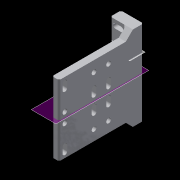
# Autodesk Inventor part: AXTS
Saved by Autodesk Inventor 2016 (Build 200138000, 138)
## iProperties
Created: 2017-07-16
Part Number: AXTS
Material: PC/ABS Plastic
Document SubType Name: Modeling
Designer: ludwi
Density: 0.357273 g/cm^3
Appearance: Smooth - White
Author: ludwi
Autodesk Inventor part; units mm, degrees
ref_plane "YZ Plane" through (0, 0, 0) normal (1, 0, 0) x (0, 1, 0)
ref_plane "XZ Plane" through (0, 0, 0) normal (0, 1, 0) x (-1, 0, 0)
ref_plane "XY Plane" through (0, 0, 0) normal (0, 0, 1) x (1, 0, 0)
sketch "Sketch1" plane through (0, 0, 0) normal (0, 0, 1) x (1, 0, 0)
  line L0 (0, 0) -> (32, 0)
  line L1 (32, 0) -> (32, -120)
  line L2 (32, -120) -> (22, -120)
  line L3 (22, -120) -> (22, -15)
  line L4 (22, -15) -> (0, -15)
  line L5 (0, -15) -> (0, 0)
  dimension "d3" = 120
  dimension "d4" = 10
  dimension "d5" = 22
  dimension "d8" = 15
  constraints: 12 end point, 4 perpendicular, 1 horizontal, 1 vertical
  measures "d3" distance of L0.end L1.end
  measures "d4" distance of L1.end L2.end
  measures "d5" horizontal distance of L0.start L2.end
  measures "d8" distance of L4.end L0.start
extrude "Extrusion1" add sketch "Sketch1" against normal blind 120
sketch "Sketch3" plane through (0, -15, 0) normal (-1, 0, 0) x (0, 0, 1)
  line L0 (-110, -97.8692) -> (-110, 18.1308) construction
  line L1 (-10, 18.1308) -> (-10, -97.8692) construction
  line L2 (-25, 8.9558) -> (-17, 8.9558) construction
  arc A0 (-17, 8.9558) -> (-17, 15.0558) centre (-17, 12.0058) ccw construction
  line L3 (-17, 15.0558) -> (-25, 15.0558) construction
  arc A1 (-25, 15.0558) -> (-25, 8.9558) centre (-25, 12.0058) ccw construction
  line L4 (-25, -94.7942) -> (-17, -94.7942) construction
  arc A2 (-17, -94.7942) -> (-17, -88.6942) centre (-17, -91.7442) ccw construction
  line L5 (-17, -88.6942) -> (-25, -88.6942) construction
  arc A3 (-25, -88.6942) -> (-25, -94.7942) centre (-25, -91.7442) ccw construction
  circle A4 centre (-25, -50.2442) radius 3.05 construction
  circle A5 centre (-25, -29.4942) radius 3.05 construction
  circle A6 centre (-95, -29.4942) radius 3.05 construction
  circle A7 centre (-95, -50.2442) radius 3.05 construction
  line L6 (-95, 15.0558) -> (-103, 15.0558) construction
  arc A8 (-103, 15.0558) -> (-103, 8.9558) centre (-103, 12.0058) ccw construction
  line L7 (-103, 8.9558) -> (-95, 8.9558) construction
  arc A9 (-95, 8.9558) -> (-95, 15.0558) centre (-95, 12.0058) ccw construction
  circle A10 centre (-67.125, 12.0058) radius 3.05 construction
  line L8 (-52.875, -32.5442) -> (-44.875, -32.5442) construction
  arc A11 (-44.875, -32.5442) -> (-44.875, -26.4442) centre (-44.875, -29.4942) ccw construction
  line L9 (-44.875, -26.4442) -> (-52.875, -26.4442) construction
  arc A12 (-52.875, -26.4442) -> (-52.875, -32.5442) centre (-52.875, -29.4942) ccw construction
  circle A13 centre (-52.875, -91.7442) radius 3.05 construction
  circle A14 centre (-52.875, 12.0058) radius 3.05 construction
  line L10 (-52.875, -53.2942) -> (-44.875, -53.2942) construction
  arc A15 (-44.875, -53.2942) -> (-44.875, -47.1942) centre (-44.875, -50.2442) ccw construction
  line L11 (-44.875, -47.1942) -> (-52.875, -47.1942) construction
  arc A16 (-52.875, -47.1942) -> (-52.875, -53.2942) centre (-52.875, -50.2442) ccw construction
  circle A17 centre (-67.125, -91.7442) radius 3.05 construction
  line L12 (-75.125, -53.2942) -> (-67.125, -53.2942) construction
  arc A18 (-67.125, -53.2942) -> (-67.125, -47.1942) centre (-67.125, -50.2442) ccw construction
  line L13 (-67.125, -47.1942) -> (-75.125, -47.1942) construction
  arc A19 (-75.125, -47.1942) -> (-75.125, -53.2942) centre (-75.125, -50.2442) ccw construction
  line L14 (-103, -94.7942) -> (-95, -94.7942) construction
  arc A20 (-95, -94.7942) -> (-95, -88.6942) centre (-95, -91.7442) ccw construction
  line L15 (-95, -88.6942) -> (-103, -88.6942) construction
  arc A21 (-103, -88.6942) -> (-103, -94.7942) centre (-103, -91.7442) ccw construction
  line L16 (-75.125, -32.5442) -> (-67.125, -32.5442) construction
  arc A22 (-67.125, -32.5442) -> (-67.125, -26.4442) centre (-67.125, -29.4942) ccw construction
  line L17 (-67.125, -26.4442) -> (-75.125, -26.4442) construction
  arc A23 (-75.125, -26.4442) -> (-75.125, -32.5442) centre (-75.125, -29.4942) ccw construction
  line L18 (0, -105) -> (0, 0) construction
  line L19 (0, 0) -> (-120, 0) construction
  line L20 (-120, -105) -> (-120, 0) construction
  line L21 (0, -105) -> (-120, -105) construction
  line L22 (0, 0) -> (0, 15) construction
  line L23 (0, 15) -> (-120, 15) construction
  line L24 (-120, 0) -> (-120, 15) construction
  line L25 (0, 0) -> (-120, 0) construction
  line L26 (-120, 0) -> (-110, -10)
  line L27 (-110, -99.8692) -> (-110, -10)
  line L28 (0, -105) -> (-120, -105) projected
  line L29 (-120, -105) -> (-110, -99.8692)
  line L30 (-120, -105) -> (-120, 0)
  line L31 (-120, 15) -> (-120, -105) projected
  line L32 (0, 0) -> (-120, 0) projected
  line L33 (0, 0) -> (-10, -10)
  line L34 (-10, -10) -> (-10, -99.8692)
  line L35 (0, 15) -> (0, -105) projected
  line L36 (-10, -99.8692) -> (0, -105)
  line L37 (0, -105) -> (0, -105)
  line L38 (0, 0) -> (0, -105)
  line L39 (-120, -98.4303) -> (-110, -98.4303)
  line L40 (-110, -98.4303) -> (-110, -107.1574)
  line L41 (-110, -107.1574) -> (-120, -107.1574)
  line L42 (-120, -107.1574) -> (-120, -98.4303)
  line L43 (0, -94.7942) -> (-10, -94.7942)
  line L44 (-10, -94.7942) -> (-10, -110)
  line L45 (-10, -110) -> (0, -110)
  line L46 (0, -110) -> (0, -94.7942)
  line L47 (-10, 18.1308) -> (-110, 18.1308) projected
  line L48 (-110, -97.8692) -> (-10, -97.8692) projected
  point P0 (-213, 15.0558)
  point P1 (-213, -88.6942)
  point P2 (-127, 8.9558)
  point P3 (-185.125, -26.4442)
  point P4 (-185.125, -47.1942)
  point P5 (-162.875, -47.1942)
  point P6 (-135, -88.6942)
  point P7 (-162.875, -26.4442)
  dimension "d3" = 120
  dimension "d4" = 10
  dimension "d5" = 22
  dimension "d8" = 15
  dimension "d12" = 135
  dimension "d13" = 135
  constraints: 34 end point, 4 parallel, 4 point on line, 3 perpendicular, 2 collinear, 2 horizontal
  measures "d12" angle of L35 L33
  measures "d13" angle of L20 L26
extrude "Extrusion2" cut sketch "Sketch3" against normal through all contours L26 L27 L39 L30 | L39 L27 L29 L30 | L35 L43 L34 L33 | L29 L40 L28 | L28 L40 L41 L42 | L35 L36 L34 L43 | L46 L45 L44 L28 | L28 L44 L36
chamfer "Chamfer2" distance 2 angle 45 6 edges at (22, -15, -60) (0, -15, -60) (0, 0, -60) (32, 0, -60) (32, -120, -60) (22, -120, -60)
sketch "Sketch4" plane through (2, -15, -120) normal (0, -1, 0) x (1, 0, 0)
  line L0 (98.1462, 2) -> (-1.8538, 2) construction
  line L1 (98.1462, 2) -> (98.1462, 118) construction
  line L2 (-1.8538, 118) -> (98.1462, 118) construction
  line L3 (-1.8538, 118) -> (-1.8538, 2) construction
  line L4 (83.1462, 11.175) -> (91.1462, 11.175) construction
  arc A0 (91.1462, 5.075) -> (91.1462, 11.175) centre (91.1462, 8.125) ccw construction
  line L5 (91.1462, 5.075) -> (83.1462, 5.075) construction
  arc A1 (83.1462, 11.175) -> (83.1462, 5.075) centre (83.1462, 8.125) ccw construction
  line L6 (83.1462, 114.925) -> (91.1462, 114.925) construction
  arc A2 (91.1462, 108.825) -> (91.1462, 114.925) centre (91.1462, 111.875) ccw construction
  line L7 (91.1462, 108.825) -> (83.1462, 108.825) construction
  arc A3 (83.1462, 114.925) -> (83.1462, 108.825) centre (83.1462, 111.875) ccw construction
  circle A4 centre (83.1462, 70.375) radius 3.05 construction
  circle A5 centre (83.1462, 49.625) radius 3.05 construction
  circle A6 centre (13.1462, 49.625) radius 3.05 construction
  circle A7 centre (13.1462, 70.375) radius 3.05 construction
  line L8 (13.1462, 5.075) -> (5.1462, 5.075) construction
  arc A8 (5.1462, 11.175) -> (5.1462, 5.075) centre (5.1462, 8.125) ccw construction
  line L9 (5.1462, 11.175) -> (13.1462, 11.175) construction
  arc A9 (13.1462, 5.075) -> (13.1462, 11.175) centre (13.1462, 8.125) ccw construction
  circle A10 centre (41.0212, 8.125) radius 3.05 construction
  line L10 (55.2712, 52.675) -> (63.2712, 52.675) construction
  arc A11 (63.2712, 46.575) -> (63.2712, 52.675) centre (63.2712, 49.625) ccw construction
  line L11 (63.2712, 46.575) -> (55.2712, 46.575) construction
  arc A12 (55.2712, 52.675) -> (55.2712, 46.575) centre (55.2712, 49.625) ccw construction
  circle A13 centre (55.2712, 111.875) radius 3.05 construction
  circle A14 centre (55.2712, 8.125) radius 3.05 construction
  line L12 (55.2712, 73.425) -> (63.2712, 73.425) construction
  arc A15 (63.2712, 67.325) -> (63.2712, 73.425) centre (63.2712, 70.375) ccw construction
  line L13 (63.2712, 67.325) -> (55.2712, 67.325) construction
  arc A16 (55.2712, 73.425) -> (55.2712, 67.325) centre (55.2712, 70.375) ccw construction
  circle A17 centre (41.0212, 111.875) radius 3.05 construction
  line L14 (33.0212, 73.425) -> (41.0212, 73.425) construction
  arc A18 (41.0212, 67.325) -> (41.0212, 73.425) centre (41.0212, 70.375) ccw construction
  line L15 (41.0212, 67.325) -> (33.0212, 67.325) construction
  arc A19 (33.0212, 73.425) -> (33.0212, 67.325) centre (33.0212, 70.375) ccw construction
  line L16 (5.1462, 114.925) -> (13.1462, 114.925) construction
  arc A20 (13.1462, 108.825) -> (13.1462, 114.925) centre (13.1462, 111.875) ccw construction
  line L17 (13.1462, 108.825) -> (5.1462, 108.825) construction
  arc A21 (5.1462, 114.925) -> (5.1462, 108.825) centre (5.1462, 111.875) ccw construction
  line L18 (33.0212, 52.675) -> (41.0212, 52.675) construction
  arc A22 (41.0212, 46.575) -> (41.0212, 52.675) centre (41.0212, 49.625) ccw construction
  line L19 (41.0212, 46.575) -> (33.0212, 46.575) construction
  arc A23 (33.0212, 52.675) -> (33.0212, 46.575) centre (33.0212, 49.625) ccw construction
  line L20 (13.1462, 49.625) -> (5.1462, 49.625) construction
  line L21 (13.1462, 46.575) -> (5.1462, 46.575) construction
  line L22 (5.1462, 52.675) -> (13.1462, 52.675) construction
  arc A24 (13.1462, 46.575) -> (13.1462, 52.675) centre (13.1462, 49.625) ccw construction
  arc A25 (5.1462, 52.675) -> (5.1462, 46.575) centre (5.1462, 49.625) ccw construction
  line L23 (13.1462, 70.375) -> (5.1462, 70.375) construction
  line L24 (13.1462, 67.325) -> (5.1462, 67.325) construction
  line L25 (5.1462, 73.425) -> (13.1462, 73.425) construction
  arc A26 (13.1462, 67.325) -> (13.1462, 73.425) centre (13.1462, 70.375) ccw construction
  arc A27 (5.1462, 73.425) -> (5.1462, 67.325) centre (5.1462, 70.375) ccw construction
  line L26 (13.1462, 111.875) -> (5.1462, 111.875) construction
  line L27 (13.1462, 108.825) -> (5.1462, 108.825) construction
  line L28 (5.1462, 114.925) -> (13.1462, 114.925) construction
  arc A28 (13.1462, 108.825) -> (13.1462, 114.925) centre (13.1462, 111.875) ccw construction
  arc A29 (5.1462, 114.925) -> (5.1462, 108.825) centre (5.1462, 111.875) ccw construction
  line L29 (13.1462, 8.125) -> (5.1462, 8.125) construction
  line L30 (13.1462, 5.075) -> (5.1462, 5.075) construction
  line L31 (5.1462, 11.175) -> (13.1462, 11.175) construction
  arc A30 (13.1462, 5.075) -> (13.1462, 11.175) centre (13.1462, 8.125) ccw construction
  arc A31 (5.1462, 11.175) -> (5.1462, 5.075) centre (5.1462, 8.125) ccw construction
  line L32 (13.1462, 11.475) -> (5.1462, 11.475)
  arc A32 (5.1462, 11.475) -> (5.1462, 4.775) centre (5.1462, 8.125) ccw
  line L33 (5.1462, 4.775) -> (13.1462, 4.775)
  arc A33 (13.1462, 4.775) -> (13.1462, 11.475) centre (13.1462, 8.125) ccw
  line L34 (13.1462, 52.975) -> (5.1462, 52.975)
  arc A34 (5.1462, 52.975) -> (5.1462, 46.275) centre (5.1462, 49.625) ccw
  line L35 (5.1462, 46.275) -> (13.1462, 46.275)
  arc A35 (13.1462, 46.275) -> (13.1462, 52.975) centre (13.1462, 49.625) ccw
  line L36 (13.1462, 73.725) -> (5.1462, 73.725)
  arc A36 (5.1462, 73.725) -> (5.1462, 67.025) centre (5.1462, 70.375) ccw
  line L37 (5.1462, 67.025) -> (13.1462, 67.025)
  arc A37 (13.1462, 67.025) -> (13.1462, 73.725) centre (13.1462, 70.375) ccw
  line L38 (13.1462, 115.225) -> (5.1462, 115.225)
  arc A38 (5.1462, 115.225) -> (5.1462, 108.525) centre (5.1462, 111.875) ccw
  line L39 (5.1462, 108.525) -> (13.1462, 108.525)
  arc A39 (13.1462, 108.525) -> (13.1462, 115.225) centre (13.1462, 111.875) ccw
  point P0 (-2, 120)
  point P1 (9.1462, 49.625)
  point P2 (9.1462, 70.375)
  point P3 (9.1462, 111.875)
  point P4 (9.1462, 8.125)
  dimension "d30" = 0.3
  constraints: 48 end point, 32 point on circle, 16 centre point, 16 tangent, 9 parallel, 5 equal radius, 4 midpoint, 1 horizontal, 12 other
  measures "d30" radial gap between concentric circles of A36 A27
sketch "Sketch5" plane through (22, -118, -10) normal (-1, 0, 0) x (0, 0, 1)
  line L0 (0, 116.1308) -> (-100, 116.1308) construction
  line L1 (0, 116.1308) -> (0, 0.1308) construction
  line L2 (-100, 0.1308) -> (0, 0.1308) construction
  line L3 (-100, 0.1308) -> (-100, 116.1308) construction
  line L4 (-15, 106.9558) -> (-7, 106.9558) construction
  arc A0 (-7, 106.9558) -> (-7, 113.0558) centre (-7, 110.0058) ccw construction
  line L5 (-7, 113.0558) -> (-15, 113.0558) construction
  arc A1 (-15, 113.0558) -> (-15, 106.9558) centre (-15, 110.0058) ccw construction
  line L6 (-15, 3.2058) -> (-7, 3.2058) construction
  arc A2 (-7, 3.2058) -> (-7, 9.3058) centre (-7, 6.2558) ccw construction
  line L7 (-7, 9.3058) -> (-15, 9.3058) construction
  arc A3 (-15, 9.3058) -> (-15, 3.2058) centre (-15, 6.2558) ccw construction
  circle A4 centre (-15, 47.7558) radius 3.05 construction
  circle A5 centre (-15, 68.5058) radius 3.05 construction
  circle A6 centre (-85, 68.5058) radius 3.05 construction
  circle A7 centre (-85, 47.7558) radius 3.05 construction
  line L8 (-85, 113.0558) -> (-93, 113.0558) construction
  arc A8 (-93, 113.0558) -> (-93, 106.9558) centre (-93, 110.0058) ccw construction
  line L9 (-93, 106.9558) -> (-85, 106.9558) construction
  arc A9 (-85, 106.9558) -> (-85, 113.0558) centre (-85, 110.0058) ccw construction
  circle A10 centre (-57.125, 110.0058) radius 3.05 construction
  line L10 (-42.875, 65.4558) -> (-34.875, 65.4558) construction
  arc A11 (-34.875, 65.4558) -> (-34.875, 71.5558) centre (-34.875, 68.5058) ccw construction
  line L11 (-34.875, 71.5558) -> (-42.875, 71.5558) construction
  arc A12 (-42.875, 71.5558) -> (-42.875, 65.4558) centre (-42.875, 68.5058) ccw construction
  circle A13 centre (-42.875, 6.2558) radius 3.05 construction
  circle A14 centre (-42.875, 110.0058) radius 3.05 construction
  line L12 (-42.875, 44.7058) -> (-34.875, 44.7058) construction
  arc A15 (-34.875, 44.7058) -> (-34.875, 50.8058) centre (-34.875, 47.7558) ccw construction
  line L13 (-34.875, 50.8058) -> (-42.875, 50.8058) construction
  arc A16 (-42.875, 50.8058) -> (-42.875, 44.7058) centre (-42.875, 47.7558) ccw construction
  circle A17 centre (-57.125, 6.2558) radius 3.05 construction
  line L14 (-65.125, 44.7058) -> (-57.125, 44.7058) construction
  arc A18 (-57.125, 44.7058) -> (-57.125, 50.8058) centre (-57.125, 47.7558) ccw construction
  line L15 (-57.125, 50.8058) -> (-65.125, 50.8058) construction
  arc A19 (-65.125, 50.8058) -> (-65.125, 44.7058) centre (-65.125, 47.7558) ccw construction
  line L16 (-93, 3.2058) -> (-85, 3.2058) construction
  arc A20 (-85, 3.2058) -> (-85, 9.3058) centre (-85, 6.2558) ccw construction
  line L17 (-85, 9.3058) -> (-93, 9.3058) construction
  arc A21 (-93, 9.3058) -> (-93, 3.2058) centre (-93, 6.2558) ccw construction
  line L18 (-65.125, 65.4558) -> (-57.125, 65.4558) construction
  arc A22 (-57.125, 65.4558) -> (-57.125, 71.5558) centre (-57.125, 68.5058) ccw construction
  line L19 (-57.125, 71.5558) -> (-65.125, 71.5558) construction
  arc A23 (-65.125, 71.5558) -> (-65.125, 65.4558) centre (-65.125, 68.5058) ccw construction
  circle A24 centre (-57.125, 6.2558) radius 3.35
  circle A25 centre (-42.875, 6.2558) radius 3.35
  circle A26 centre (-85, 47.7558) radius 3.35
  circle A27 centre (-85, 68.5058) radius 3.35
  circle A28 centre (-15, 47.7558) radius 3.35
  circle A29 centre (-15, 68.5058) radius 3.35
  line L20 (-93, 9.6058) -> (-85, 9.6058)
  arc A30 (-85, 2.9058) -> (-85, 9.6058) centre (-85, 6.2558) ccw
  line L21 (-85, 2.9058) -> (-93, 2.9058)
  arc A31 (-93, 9.6058) -> (-93, 2.9058) centre (-93, 6.2558) ccw
  line L22 (-15, 9.6058) -> (-7, 9.6058)
  arc A32 (-7, 2.9058) -> (-7, 9.6058) centre (-7, 6.2558) ccw
  line L23 (-7, 2.9058) -> (-15, 2.9058)
  arc A33 (-15, 9.6058) -> (-15, 2.9058) centre (-15, 6.2558) ccw
  line L24 (-42.875, 51.1058) -> (-34.875, 51.1058)
  arc A34 (-34.875, 44.4058) -> (-34.875, 51.1058) centre (-34.875, 47.7558) ccw
  line L25 (-34.875, 44.4058) -> (-42.875, 44.4058)
  arc A35 (-42.875, 51.1058) -> (-42.875, 44.4058) centre (-42.875, 47.7558) ccw
  line L26 (-65.125, 51.1058) -> (-57.125, 51.1058)
  arc A36 (-57.125, 44.4058) -> (-57.125, 51.1058) centre (-57.125, 47.7558) ccw
  line L27 (-57.125, 44.4058) -> (-65.125, 44.4058)
  arc A37 (-65.125, 51.1058) -> (-65.125, 44.4058) centre (-65.125, 47.7558) ccw
  line L28 (-65.125, 71.8558) -> (-57.125, 71.8558)
  arc A38 (-57.125, 65.1558) -> (-57.125, 71.8558) centre (-57.125, 68.5058) ccw
  line L29 (-57.125, 65.1558) -> (-65.125, 65.1558)
  arc A39 (-65.125, 71.8558) -> (-65.125, 65.1558) centre (-65.125, 68.5058) ccw
  line L30 (-42.875, 71.8558) -> (-34.875, 71.8558)
  arc A40 (-34.875, 65.1558) -> (-34.875, 71.8558) centre (-34.875, 68.5058) ccw
  line L31 (-34.875, 65.1558) -> (-42.875, 65.1558)
  arc A41 (-42.875, 71.8558) -> (-42.875, 65.1558) centre (-42.875, 68.5058) ccw
  point P0 (10, 118)
  dimension "d29" = 0.3
  constraints: 24 end point, 24 point on circle, 18 centre point, 11 equal radius, 6 coincident, 18 other
  measures "d29" distance between parallel lines of L28 L19
extrude "Extrusion3" cut sketch "Sketch5" against normal through all
extrude "Extrusion4" cut sketch "Sketch4" against normal through all
ref_plane "Work Plane1" through (0, 0, -35) normal (0, 0, 1) x (1, 0, 0)
sketch "Sketch6" plane through (0, 0, -35) normal (0, 0, 1) x (1, 0, 0)
  point P0 (0, 0)
sketch "Sketch7" plane through (0, 0, -35) normal (0, 0, 1) x (1, 0, 0)
  line L0 (32, -118) -> (30, -120) construction
  line L1 (30, -120) -> (24, -120) construction
  line L2 (24, -120) -> (22, -118) construction
  line L3 (22, -118) -> (22, -17) construction
  line L4 (22, -17) -> (20, -15) construction
  line L5 (20, -15) -> (2, -15) construction
  line L6 (2, -15) -> (0, -13) construction
  line L7 (0, -13) -> (0, -2) construction
  line L8 (0, -2) -> (2, 0) construction
  line L9 (2, 0) -> (30, 0) construction
  line L10 (30, 0) -> (32, -2) construction
  line L11 (32, -2) -> (32, -118) construction
  line L12 (0, -13) -> (2, -15) projected
  line L13 (2, -15) -> (22, -35)
  line L14 (22, -35) -> (22, -15)
  line L15 (32, -15) -> (20, -15) projected
  line L16 (22, -25) -> (22, -118) projected
  line L17 (22, -15) -> (2, -15)
  point P0 (0, 0)
  constraints: 6 end point, 3 collinear, 2 point on line
extrude "Extrusion5" add sketch "Sketch7" along normal blind 5
chamfer "Chamfer3" distance 2 angle 45 6 edges at (11, -15, -30) (21, -16, -30) (22, -26, -30) (11, -15, -35) (21, -16, -35) (22, -26, -35)
ref_plane "Work Plane2" through (0, 0, -60) normal (0, 0, -1) x (-1, 0, 0)
mirror "Mirror1" about plane through (0, 0, -60) normal (0, 0, -1) of "Extrusion5", "Chamfer3"
body "Solid1"
